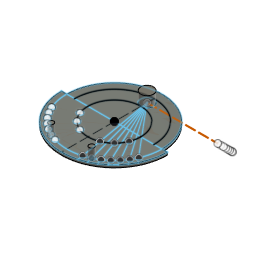
Tangible Interfaces Plate Definitive (Autodesk Fusion 360 design; units mm, degrees)
Autodesk Fusion 360 part; units mm, degrees
note: some values were not read from the file. Set by a fixed rule: which sketch regions a step uses.
sketch "Sketch1" plane through (0, 0, 0) normal (0, 1, 0) x (1, 0, 0)
  arc A0 (37.5, 0) -> (-37.5, 0) centre (0, 0) ccw
  line L0 (-37.5, 0) -> (37.5, 0)
  line L1 (-50, 0) -> (-37.5, 0)
  line L2 (50, 0) -> (37.5, 0)
  arc A1 (-50, 0) -> (50, 0) centre (0, 0) ccw
  line L3 (0, 37.5) -> (0, 31)
  circle A2 centre (0, 31) radius 6
  line L4 (0, 37.5) -> (0, -50) construction
  line L5 (0, 31) -> (20.5233, -45.5938)
  line L6 (0, 31) -> (79.2958, 31) construction
  line L7 (0, 31) -> (80.809, 31) construction
  line L8 (0, 31) -> (13.9333, -48.0194)
  line L9 (0, 31) -> (80.2384, 31) construction
  line L10 (0, 31) -> (26.6753, -42.2898)
  line L11 (0, 31) -> (77.9934, 31) construction
  line L12 (0, 31) -> (32.2663, -38.1953)
  line L13 (0, 31) -> (76.3486, 31) construction
  line L14 (0, 31) -> (37.1918, -33.4181)
  line L15 (0, 31) -> (74.3836, 31) construction
  line L16 (0, 31) -> (44.7413, -22.3207)
  line L17 (0, 31) -> (69.6052, 31) construction
  line L18 (0, 31) -> (41.3694, -28.0816)
  line L19 (0, 31) -> (72.1253, 31) construction
  line L20 (0, 31) -> (66.8592, 31) construction
  circle A3 centre (41.1995, -18.0997) radius 2.5
  circle A4 centre (38.2758, -23.6635) radius 2.5
  circle A5 centre (34.5465, -28.8364) radius 2.5
  circle A6 centre (30.0677, -33.4804) radius 2.5
  circle A7 centre (24.9208, -37.4694) radius 2.5
  circle A8 centre (19.2102, -40.6936) radius 2.5
  circle A9 centre (13.0594, -43.0634) radius 2.5
  circle A10 centre (0, 0) radius 25
  circle A11 centre (0, 0) radius 45
  circle A12 centre (9.5407, -23.1079) radius 2.5
  circle A13 centre (17.7067, -17.6486) radius 2.5
  circle A14 centre (23.2309, -9.2371) radius 2.5
  circle A15 centre (-9.5407, -23.1079) radius 2.5
  circle A16 centre (-17.7067, -17.6486) radius 2.5
  circle A17 centre (-23.2309, -9.2371) radius 2.5
  circle A18 centre (-13.0594, -43.0634) radius 2.5
  circle A19 centre (-19.2102, -40.6936) radius 2.5
  circle A20 centre (-24.9208, -37.4694) radius 2.5
  circle A21 centre (-30.0677, -33.4804) radius 2.5
  circle A22 centre (-34.5465, -28.8364) radius 2.5
  circle A23 centre (-38.2758, -23.6635) radius 2.5
  circle A24 centre (-41.1995, -18.0997) radius 2.5
  dimension "d1" = 75
  dimension "d3" = 75
  dimension "d5" = 80
  dimension "d6" = 70
  dimension "d7" = 65
  dimension "d8" = 60
  dimension "d9" = 50
  dimension "d10" = 55
  dimension "d13" = 5
  dimension "d14" = 5
  dimension "d15" = 5
  dimension "d16" = 5
  dimension "d17" = 5
  dimension "d18" = 5
  dimension "d19" = 5
  dimension "d21" = 50
  dimension "d26" = 5
  dimension "d27" = 5
  dimension "d28" = 5
  constraint coincident A0.centre A1.centre
  constraint horizontal L0
  constraint parallel L0 L1
  constraint parallel L0 L2
  constraint midpoint A0 L3.start
  constraint vertical L3
  constraint coincident L3.end A2.centre
  constraint midpoint A1 L4.end
  constraint horizontal L6
  constraint coincident A1 L5.end
  constraint horizontal L7
  constraint horizontal L9
  constraint coincident A1 L8.end
  constraint horizontal L11
  constraint coincident A1 L10.end
  constraint horizontal L13
  constraint coincident A1 L12.end
  constraint horizontal L15
  constraint coincident A1 L14.end
  constraint horizontal L17
  constraint coincident A1 L16.end
  constraint horizontal L19
  constraint coincident A1 L18.end
  constraint horizontal L20
  constraint coincident L16 A3.centre
  constraint coincident L18 A4.centre
  constraint coincident L14 A5.centre
  constraint coincident L12 A6.centre
  constraint coincident L10 A7.centre
  constraint coincident L5 A8.centre
  constraint coincident L8 A9.centre
  constraint concentric A0 A11
  constraint coincident A10 A12.centre
  constraint coincident L8 A12.centre
  constraint coincident A10 A13.centre
  constraint coincident L10 A13.centre
  constraint coincident A10 A14.centre
  constraint coincident L14 A14.centre
  constraint symmetric L4 A3 A24
  constraint symmetric L4 A4 A23
  constraint symmetric L4 A5 A22
  constraint symmetric L4 A6 A21
  constraint symmetric L4 A7 A20
  constraint symmetric L4 A8 A19
  constraint symmetric L4 A9 A18
  constraint symmetric L4 A12 A15
  constraint symmetric L4 A13 A16
  constraint symmetric L4 A14 A17
  measures "d1" diameter of A0
  measures "d3" angle of L5 L6
  measures "d5" angle of L8 L9
  measures "d6" angle of L10 L11
  measures "d7" angle of L12 L13
  measures "d8" angle of L14 L15
  measures "d9" angle of L16 L17
  measures "d10" angle of L18 L19
  measures "d13" diameter of A3
  measures "d14" diameter of A4
  measures "d15" diameter of A5
  measures "d16" diameter of A6
  measures "d17" diameter of A7
  measures "d18" diameter of A8
  measures "d19" diameter of A9
  measures "d21" diameter of A10
  measures "d26" diameter of A12
  measures "d27" diameter of A13
  measures "d28" diameter of A14
extrude "Extrude2" add sketch "Sketch1" against normal blind 2.5 makes body 1
extrude "Extrude1" add sketch "Sketch1" along normal blind 10 separate body contours L3 A2 L16 | L3 A2 L8 | A2 L5 L10 | A2 L5 L8 | A2 L10 L12 | A2 L12 L14 | A2 L14 L18 | A2 L16 L18 makes body 2
extrude "Extrude3" add sketch "Sketch1" along normal blind 10 contours L5 A8 A11 | L5 A8 A11 | L5 A8 A11 | L5 A8 A11 | A11 A19 | A11 A19 bodies 1
